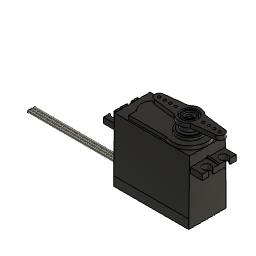
cad_components_fusion360 (Autodesk Fusion 360 archive; units mm, degrees)
design "Servo - MG 996R"
Autodesk Fusion 360 part; units mm, degrees
sketch "Sketch1" plane through (0, 0, 0) normal (1, 0, 0) x (0, 1, 0)
  line L0 (10.2, -18.25) -> (-10.2, -18.25)
  line L1 (-10.2, -18.25) -> (-10.2, -11.25)
  line L2 (-9.75, 18.25) -> (9.75, 18.25)
  line L3 (10.2, -11.25) -> (10.2, -18.25)
  line L4 (-10.2, -11.25) -> (-10.2, -18.25)
  line L5 (-10.2, -11.25) -> (-9.75, 18.25)
  line L6 (10.2, -11.25) -> (9.75, 18.25)
  line L7 (-9.3077, 9.75) -> (9.1923, 9.75)
  line L8 (9.1923, 9.75) -> (9.1923, 12.75)
  line L9 (9.1923, 12.75) -> (-9.3077, 12.75)
  line L10 (-9.3077, 12.75) -> (-9.3077, 9.75)
  line L11 (0, 18.25) -> (-0.0577, 12.75)
  dimension "d4" = 7
  dimension "d9" = 18.5
  dimension "d10" = 3
  dimension "d11" = 8.5
  constraint horizontal L0
  constraint perpendicular L0 L1
  constraint parallel L0 L2
  constraint parallel L1 L3
  constraint vertical L4
  constraint horizontal L7
  constraint vertical L8
  constraint horizontal L9
  constraint vertical L10
  constraint midpoint L2 L11.start
  constraint midpoint L9 L11.end
  measures "d4" distance of L0.end L1.end
  measures "d9" distance of L7.start L7.end
  measures "d10" distance of L7.start L9.end
  measures "d11" distance of L2 L7
extrude "Extrude1" add sketch "Sketch1" along normal mid plane 41 contours L0 L1 L2 L3 L4 L5 L6 | L7 L8 L9 L10 makes body 1
chamfer "Chamfer1" distance 2 angle 45 2 edges at (0, -10.2, -18.25) (0, 10.2, -18.25) on bodies 1
chamfer "Chamfer1" distance 2 angle 45 2 edges at (20.5, 0, -18.25) (-20.5, 0, -18.25) on bodies 1
extrude "Extrude2" add sketch "Sketch1" along normal mid plane 54 contours L7 L8 L9 L10 bodies 1
sketch "Sketch2" plane through (0, 0, 0) normal (0, 1, 0) x (1, 0, 0)
  line L0 (20.5, -9.75) -> (27, -9.75)
  line L1 (20.5, -9.75) -> (20.5, -13.45)
  line L2 (20.5, -13.45) -> (27, -12.75)
  line L3 (-20.5, -18.25) -> (20.5, -18.25)
  line L4 (0, 0) -> (0, -19)
  line L5 (0, 11.25) -> (0, -18.25)
  line L6 (-20.5, -13.45) -> (-27, -12.75)
  line L7 (-20.5, -9.75) -> (-20.5, -13.45)
  line L8 (-27, -12.75) -> (-20.5, -12.75)
  line L9 (27, -12.75) -> (20.5, -12.75)
  point P0 (20.5, -9.75)
  point P1 (27, -12.75)
  point P2 (20.5, -12.75)
  dimension "d14" = 3.7
  constraint coincident P0 L0.start
  constraint perpendicular L0 L1
  constraint coincident P1 L2.end
  constraint coincident L4.start origin
  constraint perpendicular L3 L4
  constraint symmetric P0 L5 L7.start
  constraint symmetric L1.end L5 L6.start
  constraint symmetric P1 L5 L6.end
  constraint coincident L7 L8.end
  constraint perpendicular L7 L8
  constraint coincident P2 L9.end
  measures "d14" distance of P0 L1.end
extrude "Extrude3" add sketch "Sketch2" along normal mid plane 1 bodies 1
sketch "Sketch3" plane through (0, 0, 0) normal (0, 0, 1) x (1, 0, 0)
  line L0 (27, -0.5) -> (27, -9.3077)
  line L1 (20.5, 0) -> (27, 0)
  line L2 (20.5, -9.3077) -> (27, -9.3077)
  line L3 (23.75, 0) -> (23.75, -9.3077)
  line L4 (23.75, -4.6539) -> (27, -4.6539)
  line L5 (22.6, -4.6539) -> (22.6, -6)
  line L6 (24.8, -4.6539) -> (27, -4.6539)
  line L7 (27, -5.7539) -> (26.7053, -5.7539)
  line L8 (24.8, -4.6539) -> (27, -4.6539)
  line L9 (27, -3.5539) -> (26.7053, -3.5539)
  arc A0 (26.7053, -3.5539) -> (26.7053, -5.7539) centre (24.8, -4.6539) ccw
  line L10 (27, -5.7539) -> (27, -3.5539)
  line L11 (27, 5.7539) -> (26.7053, 5.7539)
  line L12 (27, 5.7539) -> (27, 3.5539)
  line L13 (27, 3.5539) -> (26.7053, 3.5539)
  arc A1 (26.7053, 5.7539) -> (26.7053, 3.5539) centre (24.8, 4.6539) ccw
  line L14 (0, -9.75) -> (0, 9.75)
  line L15 (-27, -5.7539) -> (-26.7053, -5.7539)
  line L16 (-27, -5.7539) -> (-27, -3.5539)
  line L17 (-27, -3.5539) -> (-26.7053, -3.5539)
  arc A2 (-26.7053, -5.7539) -> (-26.7053, -3.5539) centre (-24.8, -4.6539) ccw
  line L18 (-27, 3.5539) -> (-26.7053, 3.5539)
  line L19 (-27, 5.7539) -> (-27, 3.5539)
  line L20 (-27, 5.7539) -> (-26.7053, 5.7539)
  arc A3 (-26.7053, 3.5539) -> (-26.7053, 5.7539) centre (-24.8, 4.6539) ccw
  line L21 (20, 8.9) -> (20, -8.9)
  line L22 (6.7685, -8.9) -> (-13.5, -8.9)
  line L23 (-20.5, 0) -> (20.5, 0)
  line L24 (20.5, 9.75) -> (20.5, -9.75)
  line L25 (-13.5, 8.9) -> (6.7685, 8.9)
  arc A4 (6.7685, -8.9) -> (6.7685, 8.9) centre (10.75, 0) ccw
  circle A5 centre (10.75, 0) radius 6.5
  circle A6 centre (10.75, 0) radius 5.5
  line L26 (-9, 0) -> (-15.5, 0)
  line L27 (-13.5, -8.9) -> (-13.5, -4.6904)
  line L28 (-13.5, 4.6904) -> (-13.5, 8.9)
  arc A7 (-13.5, 4.6904) -> (-13.5, -4.6904) centre (-9, 0) ccw
  circle A8 centre (10.75, 0) radius 3
  point P0 (20.5, 0)
  dimension "d17" = 4.4
  dimension "d22" = 17.8
  dimension "d24" = 13
  dimension "d25" = 11
  dimension "d26" = 34
  dimension "d27" = 13
  dimension "d28" = 36
  dimension "d38" = 6
  constraint tangent L0 A0
  constraint midpoint L1 L3.start
  constraint midpoint L2 L3.end
  constraint midpoint L3 L4.start
  constraint perpendicular L0 L4
  constraint coincident L6.start L4
  constraint coincident L5.start A0
  constraint tangent L5 A0
  constraint perpendicular L4 L5
  constraint horizontal L6
  constraint horizontal L7
  constraint coincident L6.start L8.start
  constraint symmetric L4 L6.start L8.start
  constraint coincident L0 L7.start
  constraint coincident L0 L9.start
  constraint perpendicular L9 L10
  constraint symmetric L1 L7.start L11.start
  constraint symmetric L1 L9.start L12.end
  constraint symmetric L1 L9.end L13.end
  constraint symmetric L1 A0 A1
  constraint symmetric L1 L7.end L11.end
  constraint symmetric L7.start L14 L15.start
  constraint symmetric L9.start L14 L16.end
  constraint symmetric L9.end L14 L17.end
  constraint symmetric A0 L14 A2
  constraint symmetric L7.end L14 L15.end
  constraint symmetric L11.start L14 L19.start
  constraint symmetric L11.end L14 L20.end
  constraint symmetric L12.end L14 L18.start
  constraint symmetric L13.end L14 L18.end
  constraint symmetric A1 L14 A3
  constraint horizontal L25
  constraint perpendicular L21 L25
  constraint parallel L22 L25
  constraint parallel L21 L27
  constraint concentric A4 A5
  constraint concentric A5 A6
  constraint tangent L24 A4
  constraint coincident L23 L26.start
  constraint coincident L26.start A7.centre
  constraint coincident L23 L26.end
  constraint coincident L26.end A7
  constraint collinear L27 L28
  constraint concentric A4 A8
  measures "d17" diameter of A0
  measures "d22" distance of L21.start L21.end
  measures "d24" diameter of A5
  measures "d25" diameter of A6
  measures "d26" distance of P0 L27
  measures "d27" diameter of A7
  measures "d28" distance of P0 L26.end
  measures "d38" diameter of A8
extrude "Extrude4" cut sketch "Sketch3" along normal blind 28 contours L0 L3 L4 L6 L8 L9 A0 L10 | L0 L3 L4 L6 L7 L8 A0 L10 | L3 A0 | L11 L12 L13 A1 | L15 L16 L17 A2 | L18 L19 L20 A3 bodies 1
extrude "Extrude5" add sketch "Sketch3" along normal blind 2 from surface at 18.25 contours L21 L23 A4 | L21 L23 A4 | L14 L21 L23 L25 A4 A5 | L14 L21 L22 L23 A4 A5 | L23 A5 A6 | L23 A5 A6 | L23 A6 A8 | L23 A6 A8 | L14 L22 L23 L26 L27 A7 | L14 L23 L25 L26 L28 A7 | L23 A8 | L23 A8 bodies 1
extrude "Extrude6" add sketch "Sketch3" along normal blind 1.5 from surface at 20.25 contours L23 A5 A6 | L23 A5 A6 | L23 A6 A8 | L23 A6 A8 | L23 A8 | L23 A8 bodies 1
extrude "Extrude7" add sketch "Sketch3" along normal blind 0.5 from surface at 21.75 contours L23 A6 A8 | L23 A6 A8 | L23 A8 | L23 A8 bodies 1
copy_body "Body->Comp1" bodies 1 removing the originals makes body 2 in component "main body"
extrude "Extrude1'" add sketch "Sketch3" along normal blind 4 from surface at 22.25 separate body contours L23 A8 | L23 A8 makes body 3 in component "pin"
chamfer "Chamfer1'" distance 0.5 angle 45 1 edges at (7.953, -1.0848, 26.25) on bodies 3 in component "pin"
sketch "Sketch4" plane through (0, 0, 26.25) normal (0, 0, 1) x (-1, 0, 0)
  circle A0 centre (-10.75, 0) radius 2.5
  circle A1 centre (-10.75, 0) radius 1.5
  dimension "d43" = 3
  constraint concentric A0 A1
  measures "d43" diameter of A1
extrude "Extrude2'" cut sketch "Sketch4" against normal blind 3 contours A1 bodies 3 in component "pin"
thread "Thread1" "ISO Metric profile 3.0 M3x0.5 6H" major diameter 3.086 minor diameter 2.529 pitch 0.5 angle 60 resizes the face on face at (9.2519, 0.0748, 24.25) on bodies 3 in component "pin"
sketch "Sketch5" plane through (0, 0, 26.25) normal (0, 0, 1) x (-1, 0, 0)
  circle A0 centre (-10.75, 0) radius 1.2645
  circle A1 centre (-10.75, 0) radius 2.5
  circle A2 centre (-10.75, 0) radius 4.35
  dimension "d48" = 8.7
  constraint concentric A0 A2
  measures "d48" diameter of A2
extrude "Extrude1''" add sketch "Sketch5" against normal blind 3.5 separate body contours A2 makes body 4 in component "pinwheel"
move_face "OffsetFaces1" offset 2 1 faces at (7.0422, 0.3403, 26.25) on bodies 4 in component "pinwheel"
sketch "Sketch6" plane through (0, 0, 28.25) normal (0, 0, 1) x (-1, 0, 0)
  circle A0 centre (-10.75, 0) radius 2.5
  circle A1 centre (-10.75, 0) radius 4.35
  line L0 (8.25, -4.5) -> (-29.75, 4.5) construction
  line L1 (-29.75, -4.5) -> (8.25, 4.5) construction
  line L2 (-15.1087, 3.9764) -> (-27.5482, 2.4822)
  line L3 (-15.1087, -3.9764) -> (-27.5482, -2.4822)
  circle A2 centre (-27.25, 0) radius 0.75
  circle A3 centre (-24.25, 0) radius 0.75
  circle A4 centre (-21.25, 0) radius 0.75
  circle A5 centre (-18.25, 0) radius 0.75
  circle A6 centre (-10.75, 0) radius 5.9
  arc A7 (-27.5482, 2.4822) -> (-27.5482, -2.4822) centre (-27.25, 0) ccw
  line L4 (-10.75, 0) -> (-15.1, 0)
  line L5 (-10.75, 0) -> (-10.75, 3.2314)
  arc A8 (6.0482, -2.4822) -> (6.0482, 2.4822) centre (5.75, 0) ccw
  line L6 (-6.3913, -3.9764) -> (6.0482, -2.4822)
  line L7 (-6.3913, 3.9764) -> (6.0482, 2.4822)
  circle A9 centre (-3.25, 0) radius 0.75
  circle A10 centre (-0.25, 0) radius 0.75
  circle A11 centre (2.75, 0) radius 0.75
  circle A12 centre (5.75, 0) radius 0.75
  circle A13 centre (-10.75, 0) radius 4.5
  circle A14 centre (-10.75, 0) radius 3.5
  circle A15 centre (-10.75, 0) radius 1.5
  circle A16 centre (-10.75, 0) radius 2.85
  point P0 (-10.75, 0)
  dimension "d52" = 38
  dimension "d53" = 9
  dimension "d54" = 5
  dimension "d55" = 1.5
  dimension "d58" = -3
  dimension "d59" = 0
  dimension "d61" = 11.8
  dimension "d64" = 9
  dimension "d65" = 7
  dimension "d67" = 3
  dimension "d70" = 5.7
  constraint coincident L0 P0
  constraint coincident L1 P0
  constraint coincident P0 A0.centre
  constraint coincident A2.centre L4
  constraint tangent L2 A7
  constraint symmetric L2.end L3.end L4
  constraint concentric A2 A7
  constraint coincident A6 L2.start
  constraint coincident A6 L3.start
  constraint coincident A1 L4.end
  constraint vertical L5
  constraint symmetric L2.end L5 A8.end
  constraint symmetric L3.end L5 A8.start
  constraint symmetric A2 L5 A12
  constraint symmetric A3 L5 A11
  constraint symmetric A4 L5 A10
  constraint symmetric A5 L5 A9
  constraint symmetric L2.start L5 L7.start
  constraint symmetric L3.start L5 L6.start
  constraint symmetric A7 L5 A8
  constraint concentric A13 A14
  constraint concentric A6 A15
  measures "d52" distance of L0.end L1.end
  measures "d53" distance of L1.start L0.end
  measures "d54" diameter of A7
  measures "d55" diameter of A2
  measures "d61" diameter of A6
  measures "d64" diameter of A13
  measures "d65" diameter of A14
  measures "d67" diameter of A15
  measures "d70" diameter of A16
extrude "Extrude2''" add sketch "Sketch6" against normal blind 2.3 contours L2 L3 A6 A7 | A6 | A6 A8 L6 L7 | A13 bodies 4 in component "pinwheel"
extrude "Extrude3'" add sketch "Sketch6" against normal blind 2 contours A0 L4 L5 A15 | A0 L4 L5 A15 bodies 4 in component "pinwheel"
extrude "Extrude4'" cut sketch "Sketch6" against normal blind 1 contours A0 L4 L5 A15 | A0 L4 L5 A16 | A0 L4 L5 A15 | A0 L4 L5 A16 | A1 | A13 bodies 4 in component "pinwheel"
sketch "Sketch1 (2)" plane through (0, 0, 0) normal (1, 0, 0) x (0, 1, 0) in component "main body"
  line L0 (-10.2, -16.25) -> (10.2, -16.25)
  line L1 (0, 0) -> (0, -21)
  line L2 (-3.3, -14.65) -> (3.3, -14.65)
  line L3 (3.3, -14.65) -> (3.3, -10.65)
  line L4 (3.3, -10.65) -> (-3.3, -10.65)
  line L5 (-3.3, -10.65) -> (-3.3, -14.65)
  line L6 (-3.3, -14.65) -> (3.3, -10.65) construction
  line L7 (3.3, -14.65) -> (-3.3, -10.65) construction
  line L8 (8.2, -18.25) -> (-8.2, -18.25)
  line L9 (-3, -14.35) -> (3, -14.35)
  line L10 (3, -14.35) -> (3, -10.95)
  line L11 (3, -10.95) -> (-3, -10.95)
  line L12 (-3, -10.95) -> (-3, -14.35)
  point P0 (0, -12.65)
  dimension "d73" = 6.6
  dimension "d74" = 4
  dimension "d75" = 3.6
  dimension "d79" = -0.3
  constraint coincident L1.start origin
  constraint perpendicular L0 L1
  constraint horizontal L2
  constraint perpendicular L2 L3
  constraint parallel L2 L4
  constraint parallel L3 L5
  constraint coincident L6 P0
  constraint coincident L7 P0
  constraint coincident L1 P0
  measures "d73" distance of L3.end L4.end
  measures "d74" distance of L2.end L3.end
  measures "d75" distance of L2 L8
extrude "Extrude1'''" add sketch "Sketch1 (2)" against normal blind 1 from surface at -20.5 bodies 2 in component "main body"
extrude "Extrude2'''" add sketch "Sketch1 (2)" against normal blind 4 from surface at -21.5 contours L1 L9 L10 L11 | L1 L9 L11 L12 bodies 2 in component "main body"
sketch "Sketch2 (2)" plane through (-25.5, 0, 0) normal (-1, 0, 0) x (0, -1, 0) in component "main body"
  line L0 (-3, -14.35) -> (3, -14.35)
  line L1 (3, -14.35) -> (3, -10.95)
  line L2 (3, -10.95) -> (-3, -10.95)
  line L3 (-3, -10.95) -> (-3, -14.35)
  circle A0 centre (0, -12.65) radius 0.75
  circle A1 centre (-1.5, -12.65) radius 0.75
  circle A2 centre (1.5, -12.65) radius 0.75
  point P0 (0, -12.65)
  dimension "d83" = 1.5
  dimension "d84" = 1.5
  dimension "d85" = 1.5
  constraint coincident P0 A0.centre
  measures "d83" diameter of A0
  measures "d84" diameter of A1
  measures "d85" diameter of A2
extrude "Extrude1''''" add sketch "Sketch2 (2)" along normal blind 50 separate body contours A0 | A1 | A2 makes body 5 in component "wires\\"
component "main body" placed x (1, 0, 0) y (0, 1, 0) z (0, 0, 1) at (0, 0, 0)
component "pin" placed x (1, 0, 0) y (0, 1, 0) z (0, 0, 1) at (0, 0, 0)
component "pinwheel" placed x (1, 0, 0) y (0, 1, 0) z (0, 0, 1) at (0, 0, 0)
component "wires\\" placed x (1, 0, 0) y (0, 1, 0) z (0, 0, 1) at (0, 0, 0)
equation "d12 = 54 * 0.5 mm"
